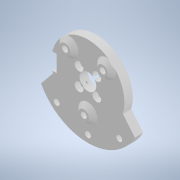
# Autodesk Inventor part: Motor_mount
Saved by Autodesk Inventor 2021 (Build 250183000, 183)
## iProperties
Created: 2026-06-06
Part Number: Motor_mount
Material: Generic
Document SubType Name: Modeling
Designer: Lukas
Density: 1 g/cm^3
Appearance: Default
Author: Lukas
Autodesk Inventor part; units mm, degrees
ref_plane "YZ Plane" through (0, 0, 0) normal (1, 0, 0) x (0, 1, 0)
ref_plane "XZ Plane" through (0, 0, 0) normal (0, 1, 0) x (-1, 0, 0)
ref_plane "XY Plane" through (0, 0, 0) normal (0, 0, 1) x (1, 0, 0)
sketch "Sketch1" plane through (0, 0, 0) normal (0, 0, 1) x (1, 0, 0)
  circle A0 centre (0, 0) radius 17.5
  arc A1 (-22.5, -12) -> (22.5, -12) centre (0, 0) ccw
  line L0 (-22.5, -12) -> (-16.7705, -5)
  line L1 (22.5, -12) -> (16.7705, -5)
  circle A2 centre (0, 0) radius 4
  circle A3 centre (-4.25, 4.25) radius 1.2
  circle A4 centre (4.25, 4.25) radius 1.2
  circle A5 centre (4.25, -4.25) radius 1.2
  circle A6 centre (-4.25, -4.25) radius 1.2
  circle A7 centre (-9, 10) radius 1.4
  circle A8 centre (9, 10) radius 1.4
  circle A9 centre (0, -13) radius 1.4
  circle A10 centre (-9, 10) radius 2.5
  circle A11 centre (9, 10) radius 2.5
  circle A12 centre (0, -13) radius 2.5
  circle A13 centre (0, -22) radius 1.4
  circle A14 centre (15, -16.0935) radius 1.4
  circle A15 centre (-15, -16.0935) radius 1.4
  line L2 (-19, 4) -> (-15, 4)
  line L3 (-15, 4) -> (-15, -4)
  line L4 (-15, -4) -> (-19, -4)
  line L5 (-19, -4) -> (-19, 4)
  point P0 (-15, 0)
  point P1 (-17.8253, -4)
  point P2 (-17.0367, 4)
  point P3 (-17.0367, -4)
  dimension "d0" = 35
  dimension "d1" = 8
  dimension "d6" = 8
  dimension "d7" = 2.4
  dimension "d8" = 8.5
  dimension "d9" = 8.5
  dimension "d10" = 4.25
  dimension "d11" = 4.25
  dimension "d12" = 23
  dimension "d13" = 18
  dimension "d14" = 2.8
  dimension "d15" = 5
  dimension "d16" = 13
  dimension "d17" = 9
  dimension "d27" = 12
  dimension "d28" = 5
  dimension "d29" = 22
  dimension "d30" = 2.8
  dimension "d32" = 15
  dimension "d33" = 22
  dimension "d34" = 22
  dimension "d35" = 15
  dimension "d36" = 4
  dimension "d37" = 8
  constraints: 16 centre point, 12 end point, 9 equal radius, 7 coincident, 7 horizontal alignment, 4 point on circle, 4 vertical alignment, 2 parallel, 1 horizontal, 1 midpoint, 1 perpendicular
  measures "d0" diameter of A0
  measures "d1" radial gap between concentric circles of A0 A1
  measures "d6" diameter of A2
  measures "d7" diameter of A4
  measures "d8" distance of A4.centre A3.centre
  measures "d9" distance of A6.centre A3.centre
  measures "d10" horizontal distance of point (0, 0) A3.centre
  measures "d11" horizontal distance of A3.centre point (0, 0)
  measures "d12" vertical distance of A8.centre A9.centre
  measures "d13" distance of A8.centre A7.centre
  measures "d14" diameter of A7
  measures "d15" diameter of A10
  measures "d16" distance of A12.centre A0.centre
  measures "d17" horizontal distance of A7.centre point (0, 0)
  measures "d27" vertical distance of A0.centre L0.start
  measures "d28" vertical distance of point (0, 0) L0.end
  measures "d29" distance of A13.centre point (0, 0)
  measures "d30" diameter of A13
  measures "d32" horizontal distance of A13.centre A15.centre
  measures "d33" distance of A1.centre A14.centre
  measures "d34" distance of A0.centre A15.centre
  measures "d35" distance from line of A0.centre L3
  measures "d36" distance of L2.start L2.end
  measures "d37" distance of L2.end L3.end
extrude "Extrusion1" add sketch "Sketch1" along normal blind 4 contours A0 L4 L3 L2 | A0 L1 A1 L0 | A10 | A11 | A12 picked at (9.375, 0)
sketch "Sketch2" plane through (0, 0, 4) normal (0, 0, 1) x (1, 0, 0)
  circle A0 centre (-4.25, 4.25) radius 1.2 projected
  circle A1 centre (-4.25, 4.25) radius 1.2 projected
  circle A2 centre (-4.25, -4.25) radius 1.2 projected
  circle A3 centre (-4.25, -4.25) radius 1.2 projected
  circle A4 centre (4.25, -4.25) radius 1.2 projected
  circle A5 centre (4.25, -4.25) radius 1.2 projected
  circle A6 centre (4.25, 4.25) radius 1.2 projected
  circle A7 centre (4.25, 4.25) radius 1.2 projected
  circle A8 centre (-4.25, 4.25) radius 2.1
  circle A9 centre (4.25, 4.25) radius 2.1
  circle A10 centre (4.25, -4.25) radius 2.1
  circle A11 centre (-4.25, -4.25) radius 2.1
  point P0 (0, 0)
  dimension "d18" = 4.2
  constraints: 4 centre point, 4 coincident, 3 equal radius
  measures "d18" diameter of A8
extrude "Extrusion2" cut sketch "Sketch2" against normal blind 2.5
sketch "Sketch3" plane through (0, 0, 4) normal (0, 0, 1) x (1, 0, 0)
  circle A0 centre (-9, 10) radius 1.4 projected
  circle A1 centre (-9, 10) radius 1.4 projected
  circle A2 centre (0, -13) radius 1.4 projected
  circle A3 centre (0, -13) radius 1.4 projected
  circle A4 centre (9, 10) radius 1.4 projected
  circle A5 centre (9, 10) radius 1.4 projected
  circle A6 centre (-9, 10) radius 2.5
  circle A7 centre (9, 10) radius 2.5
  circle A8 centre (0, -13) radius 2.5
  point P0 (0, 0)
  dimension "d21" = 5
  constraints: 3 centre point, 3 coincident, 2 equal radius
  measures "d21" diameter of A6
extrude "Extrusion3" add sketch "Sketch3" along normal blind 2
chamfer "Chamfer1" distance 2 angle 45 3 edges at (-11.5, 10, 4) (-2.5, -13, 4) (6.5, 10, 4)
sketch "Sketch4" plane through (0, 0, 4) normal (0, 0, 1) x (1, 0, 0)
  circle A0 centre (0, 0) radius 4 projected
  circle A1 centre (0, 0) radius 16.5
  line L0 (-4.2705, -15.9378) -> (-5.047, -18.8356)
  line L1 (5.047, -18.8356) -> (4.2705, -15.9378)
  arc A2 (-5.047, -18.8356) -> (5.047, -18.8356) centre (0, 0) ccw
  point P0 (0, -22)
  dimension "d38" = 33
  dimension "d41" = 30
  dimension "d42" = 3
  constraints: 4 end point, 4 point on circle, 2 centre point, 2 coincident, 2 point on line, 1 horizontal alignment, 1 vertical alignment
  measures "d38" diameter of A1
  measures "d41" angle of L1 L0
  measures "d42" radial gap between concentric circles of A1 A2
extrude "Extrusion4" cut sketch "Sketch4" along normal blind 2 contours A1 L1 A2 L0
equation "\"d9\" = d8"
equation "\"d10\" = 0.5 * d8"
equation "\"d11\" = 0.5 * d9"
equation "\"d17\" = 0.5 * d13"
equation "\"d33\" = d29"
equation "\"d34\" = d29"
body "Solid1"
